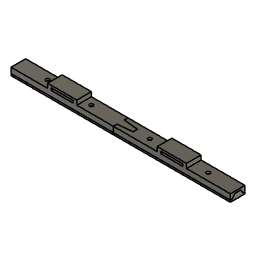
PoolHolderFinal (Autodesk Fusion 360 design; units mm, degrees)
Autodesk Fusion 360 part; units mm, degrees
note: some values were not read from the file. Chosen so that the rebuilt part matches the saved one: which bodies a step acts on; which face or edge a step refers to.
sketch "Skizze1" plane through (0, 0, 0) normal (0, 0, 1) x (1, 0, 0)
  line L0 (-75, 30) -> (225, 30)
  line L1 (225, 30) -> (225, 50)
  line L2 (225, 50) -> (-75, 50)
  line L3 (-75, 50) -> (-75, 30)
  line L4 (75, 55) -> (75, 25) construction
  dimension "d7" = 300
  dimension "d8" = 20
  constraint horizontal L0
  constraint vertical L1
  constraint horizontal L2
  constraint vertical L3
  constraint perpendicular L0 L4
  measures "d7" distance of L1.end L2.end
  measures "d8" distance of L0.start L2.end
extrude "Extrusion1" add sketch "Skizze1" along normal blind 10 makes body 1
sketch "Skizze6" plane through (0, 30, 0) normal (0, -1, 0) x (1, 0, 0)
  line L0 (-75, 0) -> (225, 0)
  line L1 (225, 0) -> (225, 10)
  line L2 (225, 10) -> (-75, 10)
  line L3 (-75, 10) -> (-75, 0)
  line L4 (-75, 10) -> (-75, 0) construction
  line L5 (-75, 5) -> (225, 5) construction
  dimension "d21" = 10
  dimension "d22" = 5
  constraint coincident L2.end L3.start
  constraint coincident L0.start L3.end
  constraint midpoint L4 L5.start
  constraint midpoint L1 L5.end
  measures "d21" distance of L2.end L0.start
  measures "d22" distance of L0 L5
sketch "Skizze8" plane through (-75, 0, 0) normal (-1, 0, 0) x (0, -1, 0)
  line L0 (-50, 0) -> (-30, 0)
  line L1 (-30, 0) -> (-30, 10)
  line L2 (-30, 10) -> (-50, 10)
  line L3 (-50, 10) -> (-50, 0)
  line L4 (-50, 5) -> (-30, 5) construction
  line L5 (-44, 7.5) -> (-36, 7.5)
  line L6 (-47.5, 2.5) -> (-44, 7.5)
  line L7 (-36, 7.5) -> (-32.5, 2.5)
  line L8 (-30, 2.5) -> (-32.5, 2.5)
  line L9 (-47.5, 2.5) -> (-50, 2.5)
  constraint midpoint L3 L4.start
  constraint midpoint L1 L4.end
  constraint perpendicular L3 L5
  constraint coincident L1 L8.start
  constraint perpendicular L1 L8
  constraint coincident L3 L9.end
  constraint perpendicular L3 L9
sketch "Skizze9" plane through (0, 0, 10) normal (0, 0, 1) x (-1, 0, 0)
  line L0 (75, -50) -> (75, -30)
  line L1 (75, -30) -> (-225, -30)
  line L2 (-225, -30) -> (-225, -50)
  line L3 (-225, -50) -> (75, -50)
  line L4 (-75, -50) -> (-75, -30) construction
  line L5 (-85, -43) -> (-85, -37)
  line L6 (-85, -43) -> (-65, -45)
  line L7 (-65, -45) -> (-65, -50)
  line L8 (-85, -37) -> (-65, -35)
  line L9 (-65, -35) -> (-65, -30)
  constraint midpoint L3 L4.start
  constraint midpoint L1 L4.end
  constraint perpendicular L3 L5
  constraint coincident L3 L7.end
  constraint perpendicular L3 L7
  constraint coincident L1 L9.end
  constraint perpendicular L1 L9
split "Teilen1" by curves path "Skizze9" along L7 L6 L5 L8 L9 bodies 1 makes body 2 at (178.3333, 39, 0)
split "Teilen2" by curves path "Skizze8" along L9 L6 L5 L7 L8 bodies 2 1 makes body 3 at (-28.3333, 38.3333, 10) makes body 4 at (178.3333, 39, 10)
extrude "Extrusion3" cut 4 faces at (65, 45.8333, 2.8571) (65, 48.3333, 6.1905) (65, 34.1667, 2.8571) (65, 31.6667, 6.1905) along direction (-1, 0, 0) blind 0.1 on bodies 1 3 bodies 1 3
extrude "Extrusion4" cut 2 faces at (75, 36, 2.5) (68.3333, 35.3333, 7.8571) along direction (-0.099504, 0.995037, 0) blind 0.1 on bodies 1 3 bodies 1 3
extrude "Extrusion5" cut 2 faces at (75, 44, 2.5) (68.3333, 44.6667, 7.8571) along direction (-0.099504, -0.995037, 0) blind 0.1 on bodies 1 3 bodies 1 3
extrude "Extrusion6" cut 2 faces at (85, 41, 2.5) (85, 41, 8.3333) along direction (-1, 0, 0) blind 0.1 on bodies 1 3 bodies 1 3
extrude "Extrusion7" cut 2 faces at (-25.335, 41.3333, 7.5) (178.3333, 41, 7.5) along direction (0, 0, -1) blind 0.1 on bodies 1 2 bodies 1 2
extrude "Extrusion8" cut 4 faces at (171.6667, 48.3333, 2.5) (-28.3667, 49.1667, 2.5) (171.6667, 30.8333, 2.5) (18.2667, 30.8333, 2.5) along direction (0, 0, -1) blind 0.1 on bodies 1 2 bodies 1 2
extrude "Extrusion9" cut 2 faces at (121.6667, 46.3333, 4.1667) (-28.3667, 45.5, 5.3571) along direction (0, -0.819232, -0.573462) blind 0.1 on bodies 1 2 bodies 1 2
extrude "Extrusion10" cut 2 faces at (121.6667, 33.6667, 4.1667) (-28.3667, 34.5, 5.3571) along direction (0, 0.819232, -0.573462) blind 0.1 on bodies 1 2 bodies 1 2
sketch "Skizze10" plane through (0, 0, 10) normal (0, 0, 1) x (-1, 0, 0)
  line L0 (-84.9, -37.0905) -> (-84.9, -42.9095)
  line L1 (-84.9, -42.9095) -> (-64.9901, -44.9005)
  line L2 (-64.9901, -44.9005) -> (-65, -45)
  line L3 (-65, -45) -> (-64.9, -45)
  line L4 (-64.9, -45) -> (-64.9, -50)
  line L5 (-64.9, -50) -> (75, -50)
  line L6 (75, -50) -> (75, -30)
  line L7 (75, -30) -> (-64.9, -30)
  line L8 (-64.9, -30) -> (-64.9, -35)
  line L9 (-64.9, -35) -> (-65, -35)
  line L10 (-65, -35) -> (-64.9901, -35.0995)
  line L11 (-64.9901, -35.0995) -> (-84.9, -37.0905)
  line L12 (75, -40) -> (-225, -40) construction
  circle A0 centre (35, -40) radius 2.55
  circle A1 centre (-24.9, -40) radius 2.55
  circle A2 centre (-104.9, -40) radius 2.55
  circle A3 centre (-185, -40) radius 2.55
  line L13 (-225, -30) -> (-225, -50) construction
  dimension "d39" = 5.1
  dimension "d40" = 5.1
  dimension "d41" = 5.1
  dimension "d42" = 5.1
  dimension "d43" = 139.9
  dimension "d44" = 140.1
  dimension "d45" = 40
  dimension "d46" = 40
  dimension "d48" = 40
  dimension "d49" = 59.9
  dimension "d51" = 80.1
  constraint midpoint L6 L12.start
  constraint perpendicular L8 L12
  constraint coincident L12 A0.centre
  constraint coincident L12 A1.centre
  constraint coincident L12 A2.centre
  constraint coincident L12 A3.centre
  measures "d39" diameter of A0
  measures "d40" diameter of A1
  measures "d41" diameter of A2
  measures "d42" diameter of A3
  measures "d43" distance of L4.end L5.end
  measures "d44" distance of L0 L13
  measures "d45" distance of L6 A0.centre
  measures "d46" distance of L4 A1.centre
  measures "d48" distance of A3.centre L13
  measures "d49" distance of A0.centre A1.centre
  measures "d51" distance of A2.centre A3.centre
extrude "Extrusion11" cut sketch "Skizze10" against normal blind 15 contours A0 | A1 | A2 | A3 bodies 1 2 3 4
sketch "Skizze11" plane through (0, 0, 10) normal (0, 0, 1) x (-1, 0, 0)
  circle A0 centre (-24.9, -40) radius 2.55
  circle A1 centre (35, -40) radius 2.55
  line L0 (-84.9, -37.0905) -> (-84.9, -42.9095)
  line L1 (-84.9, -42.9095) -> (-64.9901, -44.9005)
  line L2 (-64.9901, -44.9005) -> (-65, -45)
  line L3 (-65, -45) -> (-64.9, -45)
  line L4 (-64.9, -45) -> (-64.9, -50)
  line L5 (-64.9, -50) -> (75, -50)
  line L6 (75, -50) -> (75, -30)
  line L7 (75, -30) -> (-64.9, -30)
  line L8 (-64.9, -30) -> (-64.9, -35)
  line L9 (-64.9, -35) -> (-65, -35)
  line L10 (-65, -35) -> (-64.9901, -35.0995)
  line L11 (-64.9901, -35.0995) -> (-84.9, -37.0905)
  line L12 (35, -40) -> (-24.9, -40) construction
  line L13 (-9.95, -45) -> (-9.95, -35)
  line L14 (20.05, -35) -> (20.05, -45)
  line L15 (5.05, -35) -> (5.05, -30) construction
  line L16 (20.05, -40) -> (35, -40) construction
  line L17 (-14.95, -50) -> (-14.95, -30)
  line L18 (25.05, -30) -> (25.05, -50)
  line L19 (5.05, -50) -> (5.05, -45) construction
  line L20 (20.05, -40) -> (25.05, -40) construction
  line L21 (-9.95, -40) -> (-14.95, -40) construction
  line L22 (-9.95, -35) -> (-10, -35)
  line L23 (-10, -35) -> (-10, -30)
  line L24 (5.05, -30) -> (20.05, -30)
  line L25 (20.05, -30) -> (20.05, -35)
  line L26 (20, -50) -> (-9.95, -50)
  line L27 (-9.95, -50) -> (-9.95, -45)
  line L28 (25.05, -50) -> (20, -50)
  line L29 (-9.95, -50) -> (-14.95, -50)
  line L30 (-14.95, -30) -> (5.05, -30)
  line L31 (20.05, -30) -> (25.05, -30)
  line L32 (20.05, -45) -> (20.05, -50)
  dimension "d54" = 59.9
  dimension "d55" = 30
  dimension "d56" = 10
  dimension "d57" = 14.95
  dimension "d58" = 14.95
  dimension "d59" = 40
  dimension "d60" = 20
  dimension "d67" = 5
  dimension "d78" = 5
  constraint coincident A1.centre L12.start
  constraint coincident A0.centre L12.end
  constraint vertical L14
  constraint perpendicular L12 L13
  constraint midpoint L7 L15.end
  constraint vertical L15
  constraint midpoint L14 L16.start
  constraint horizontal L16
  constraint horizontal L28
  constraint vertical L17
  constraint horizontal L30
  constraint vertical L18
  constraint midpoint L18 L20.end
  constraint midpoint L13 L21.start
  constraint midpoint L17 L21.end
  constraint horizontal L21
  constraint vertical L19
  constraint horizontal L22
  constraint vertical L23
  constraint horizontal L24
  constraint vertical L25
  constraint coincident L23.end L30
  constraint horizontal L26
  constraint vertical L27
  constraint collinear L28 L29
  constraint collinear L30 L31
  constraint vertical L32
  measures "d54" distance of A1.centre A0.centre
  measures "d55" distance of L14.end L13.start
  measures "d56" distance of L14.end L14.start
  measures "d57" distance of A0.centre L13
  measures "d58" distance of A1.centre L14
  measures "d59" distance of L18.end L17.start
  measures "d60" distance of L18.end L18.start
  measures "d67" distance of L14.end L32.end
  measures "d78" distance of L14 L18
extrude "Extrusion14" add sketch "Skizze11" along normal blind 3 contours L5 L7 L13 L17 L22 L23 L27 L29 L30 | L5 L7 L14 L18 L25 L28 L31 L32 bodies 3
extrude "Extrusion15" add 1 faces at (-23.3833, 41.6667, 13) along direction (0, 0, 1) blind 3 on bodies 3 bodies 3
sketch "Skizze13" plane through (-20.05, 0, 0) normal (1, 0, 0) x (0, 1, 0)
  line L0 (30, 10) -> (45, 10)
  line L1 (45, 10) -> (45, 16)
  line L2 (45, 16) -> (30, 16)
  line L3 (30, 16) -> (30, 10)
  line L4 (30, 13) -> (45, 13)
  constraint midpoint L3 L4.start
  constraint midpoint L1 L4.end
extrude "Extrusion16" add sketch "Skizze13" along normal blind 35 contours L1 L2 L3 L4 bodies 3
extrude "Extrusion17" add 1 faces at (1.6167, 45, 15) along direction (0, 1, 0) blind 5 on bodies 3 bodies 3
sketch "Skizze14" plane through (0, 0, 10) normal (0, 0, 1) x (-1, 0, 0)
  circle A0 centre (-104.9, -40) radius 2.55
  circle A1 centre (-185, -40) radius 2.55
  line L0 (-65, -35) -> (-65, -30)
  line L1 (-65, -30) -> (-225, -30)
  line L2 (-225, -30) -> (-225, -50)
  line L3 (-225, -50) -> (-65, -50)
  line L4 (-65, -50) -> (-65, -45)
  line L5 (-65, -45) -> (-85, -43)
  line L6 (-85, -43) -> (-85, -37)
  line L7 (-85, -37) -> (-65, -35)
  line L8 (-225, -40) -> (-85, -40) construction
  line L9 (-104.9, -40) -> (-185, -40) construction
  line L10 (-144.95, -40) -> (-145, -50) construction
  line L11 (-144.95, -40) -> (-145, -30) construction
  line L12 (-129.95, -50) -> (-159.95, -50)
  line L13 (-159.95, -50) -> (-159.95, -30)
  line L14 (-159.95, -30) -> (-129.95, -30)
  line L15 (-129.95, -30) -> (-129.95, -50)
  line L16 (-144.95, -50) -> (-145, -50) construction
  line L17 (-159.95, -40) -> (-185, -40) construction
  line L18 (-144.95, -30) -> (-144.95, -40) construction
  line L19 (-124.95, -50) -> (-124.95, -30)
  line L20 (-164.95, -50) -> (-164.95, -30)
  dimension "d76" = 30
  dimension "d77" = 20
  dimension "d79" = 5
  dimension "d80" = 5
  constraint midpoint L2 L8.start
  constraint midpoint L6 L8.end
  constraint coincident A0.centre L9.start
  constraint coincident A1.centre L9.end
  constraint midpoint L9 L10.start
  constraint midpoint L3 L10.end
  constraint midpoint L1 L11.end
  constraint horizontal L12
  constraint vertical L13
  constraint horizontal L14
  constraint vertical L15
  constraint midpoint L12 L16.start
  constraint midpoint L13 L17.start
  constraint horizontal L16
  constraint midpoint L14 L18.start
  constraint vertical L18
  constraint coincident L3 L19.start
  constraint coincident L1 L19.end
  constraint perpendicular L1 L19
  constraint coincident L3 L20.start
  constraint coincident L1 L20.end
  constraint perpendicular L1 L20
  measures "d76" distance of L12.start L12.end
  measures "d77" distance of L12.start L14.end
  measures "d79" distance of L15 L19
  measures "d80" distance of L13 L20
extrude "Extrusion18" add sketch "Skizze14" along normal blind 6 contours L1 L3 L15 L19 | L1 L3 L13 L20 bodies 4
sketch "Skizze15" plane through (129.95, 0, 0) normal (1, 0, 0) x (0, 1, 0)
  line L0 (30, 10) -> (50, 10)
  line L1 (50, 10) -> (50, 16)
  line L2 (50, 16) -> (30, 16)
  line L3 (30, 16) -> (30, 10)
  line L4 (30, 13) -> (50, 13)
  constraint midpoint L3 L4.start
  constraint midpoint L1 L4.end
extrude "Extrusion19" add sketch "Skizze15" along normal blind 30 contours L1 L2 L3 L4 bodies 4
